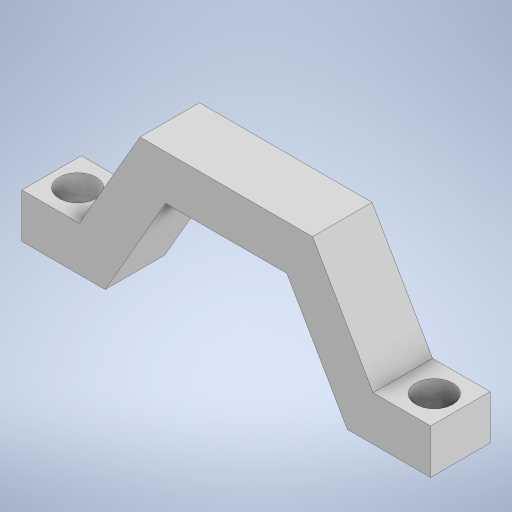
# Autodesk Inventor part: 카스벨브 하단 커버
Saved by Autodesk Inventor 2023.1 (Build 271208000, 208)
## iProperties
Created: 2022-08-17
Part Number: 카스벨브 하단 커버
Material: 일반
Document SubType Name: Modeling
Designer: fly01
Density: 1 g/cm^3
Appearance: 기본값
Author: fly01
Autodesk Inventor part; units mm, degrees
ref_plane "YZ Plane" through (0, 0, 0) normal (1, 0, 0) x (0, 1, 0)
ref_plane "XZ Plane" through (0, 0, 0) normal (0, 1, 0) x (-1, 0, 0)
ref_plane "XY Plane" through (0, 0, 0) normal (0, 0, 1) x (1, 0, 0)
sketch "스케치1" plane through (0, 0, 0) normal (0, 0, 1) x (1, 0, 0)
  line L0 (-13.75, 0) -> (13.75, 0)
  line L1 (-8.15, 0) -> (-4.075, 7.0581)
  line L2 (-4.075, 7.0581) -> (4.075, 7.0581)
  line L3 (4.075, 7.0581) -> (8.15, 0)
  line L4 (8.15, 0) -> (4.075, -7.0581)
  line L5 (4.075, -7.0581) -> (-4.075, -7.0581)
  line L6 (-4.075, -7.0581) -> (-8.15, 0)
  line L7 (-5.8071, 10.0581) -> (-11.6141, 0)
  line L8 (-11.6141, 0) -> (-5.8071, -10.0581)
  line L9 (-5.8071, -10.0581) -> (5.8071, -10.0581)
  line L10 (5.8071, -10.0581) -> (11.6141, 0)
  line L11 (11.6141, 0) -> (5.8071, 10.0581)
  line L12 (5.8071, 10.0581) -> (-5.8071, 10.0581)
  line L13 (-13.75, 0) -> (-13.75, 3)
  line L14 (-13.75, 3) -> (-9.8821, 3)
  line L15 (13.75, 0) -> (13.75, 3)
  line L16 (13.75, 3) -> (9.8821, 3)
  point P0 (0, 0)
  point P1 (0, 0)
  point P2 (0, 0)
  point P3 (8.15, 0)
  dimension "d0" = 27.5
  dimension "d1" = 16.3
  dimension "d2" = 3
  dimension "d3" = 3
  dimension "d4" = 3
  constraints: 34 end point, 3 point on line, 2 coincident, 2 perpendicular, 2 vertical, 1 horizontal, 1 midpoint, 18 other
  measures "d0" distance of L0.end L0.start
  measures "d1" distance of L3.end L1.start
  measures "d2" distance between parallel lines of L1 L7
  measures "d3" distance of L0.start L13.end
  measures "d4" distance of L0.end L15.end
extrude "돌출1" add sketch "스케치1" along normal mid plane 4 contours L13 L14 L7 L0 | L7 L12 L11 L0 L3 L2 L1 | L11 L16 L15 L0
sketch "스케치2" plane through (-13.75, 3, 2) normal (0, 1, 0) x (1, 0, 0)
  line L0 (1.75, -6.7825) -> (25.75, -6.7825)
  line L1 (25.75, -6.7825) -> (25.75, 6.7825) construction
  line L2 (25.75, 6.7825) -> (1.75, 6.7825)
  line L3 (1.75, 6.7825) -> (1.75, -6.7825) construction
  line L4 (9.675, 0) -> (17.825, 0) projected
  line L5 (1.75, -6.7825) -> (25.75, 6.7825) construction
  line L6 (25.75, -6.7825) -> (1.75, 6.7825) construction
  circle A0 centre (1.75, 2) radius 1.25
  circle A1 centre (25.75, 2) radius 1.25
  line L7 (0, 4) -> (3.8679, 4) projected
  point P0 (13.75, 2)
  point P1 (13.75, 0)
  dimension "d7" = 24
  dimension "d8" = 2.5
  dimension "d9" = 2.5
  dimension "d10" = 2
  constraints: 12 end point, 3 midpoint, 2 centre point, 2 parallel, 2 point on line, 1 horizontal, 1 horizontal alignment, 1 perpendicular
  measures "d7" distance of L1.end L2.end
  measures "d8" diameter of A0
  measures "d9" diameter of A1
  measures "d10" distance from line of L7 A0.centre
extrude "돌출2" cut sketch "스케치2" against normal blind 4
